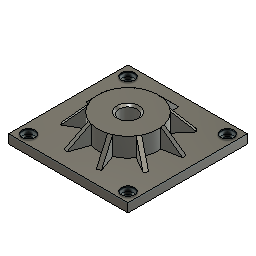
camera_mount (Autodesk Fusion 360 design; units mm, degrees)
Autodesk Fusion 360 part; units mm, degrees
sketch "Sketch1" plane through (0, 0, 0) normal (0, 1, 0) x (1, 0, 0)
  circle A0 centre (0, 0) radius 1.75
  circle A1 centre (50, 0) radius 1.75
  circle A2 centre (0, -50) radius 1.75
  circle A3 centre (50, -50) radius 1.75
  circle A4 centre (25, -25) radius 4.5
  line L0 (-5, 5) -> (55, 5)
  line L1 (55, 5) -> (55, -55)
  line L2 (55, -55) -> (-5, -55)
  line L3 (-5, -55) -> (-5, 5)
  dimension "d1" = 50
  dimension "d2" = 50
  dimension "d3" = 3.5
  dimension "d4" = 3.5
  dimension "d5" = 3.5
  dimension "d6" = 3.5
  dimension "d7" = 9
  constraint coincident A0.centre origin
  constraint horizontal L0
  constraint vertical L1
  constraint horizontal L2
  constraint vertical L3
  measures "d1" distance of A0.centre A2.centre
  measures "d2" distance of A0.centre A1.centre
  measures "d3" diameter of A0
  measures "d4" diameter of A1
  measures "d5" diameter of A2
  measures "d6" diameter of A3
  measures "d7" diameter of A4
extrude "Extrude1" add sketch "Sketch1" along normal blind 4 contours A4 | L0 L1 L2 L3
sketch "Sketch2" plane through (0, 4, 0) normal (0, 1, 0) x (-1, 0, 0)
  circle A0 centre (0, 0) radius 1.75
  circle A1 centre (-50, 0) radius 1.75
  circle A2 centre (0, 50) radius 1.75
  circle A3 centre (-50, 50) radius 1.75
  line L0 (5, 55) -> (-55, 55)
  line L1 (-55, 55) -> (-55, -5)
  line L2 (-55, -5) -> (5, -5)
  line L3 (5, -5) -> (5, 55)
  circle A4 centre (0, 0) radius 3.25
  circle A5 centre (-50, 0) radius 3.25
  circle A6 centre (0, 50) radius 3.25
  circle A7 centre (-50, 50) radius 3.25
  dimension "d10" = 6.5
  dimension "d11" = 6.5
  dimension "d12" = 6.5
  dimension "d13" = 6.5
  constraint concentric A0 A4
  constraint concentric A1 A5
  constraint concentric A2 A6
  constraint concentric A3 A7
  measures "d10" diameter of A4
  measures "d11" diameter of A5
  measures "d12" diameter of A6
  measures "d13" diameter of A7
extrude "Extrude2" add sketch "Sketch2" along normal blind 0.5 contours L0 L1 L2 L3
extrude "Extrude3" cut 1 faces at (-2.7314, 4, -0.2484) along direction (0, -1, 0) blind 2
extrude "Extrude4" cut 1 faces at (-2.7314, 4, 49.7516) along direction (0, -1, 0) blind 2
sketch "Sketch3" plane through (0, 4, 0) normal (0, 1, 0) x (-1, 0, 0)
  circle A0 centre (-50, 0) radius 3.25
  circle A1 centre (-50, 0) radius 1.75
extrude "Extrude5" cut sketch "Sketch3" against normal blind 2
extrude "Extrude6" cut 1 faces at (47.2686, 4, 49.7516) along direction (0, -1, 0) blind 2
sketch "Sketch4" plane through (0, 4.5, 0) normal (0, 1, 0) x (-1, 0, 0)
  circle A0 centre (-50, 50) radius 3.25
  circle A1 centre (-50, 0) radius 3.25
  circle A2 centre (0, 50) radius 3.25
  circle A3 centre (0, 0) radius 3.25
  line L0 (5, -5) -> (5, 55)
  line L1 (5, 55) -> (-55, 55)
  line L2 (-55, 55) -> (-55, -5)
  line L3 (-55, -5) -> (5, -5)
  line L4 (-24, 3) -> (-26, 3)
  line L5 (-10.0926, 8.7898) -> (-11.6247, 7.5042)
  line L6 (-3.1606, 22.1645) -> (-3.5079, 20.1949)
  line L7 (-6.4474, 36.866) -> (-5.4474, 35.134)
  line L8 (-18.4152, 46.0153) -> (-16.5359, 45.3312)
  line L9 (-33.4641, 45.3312) -> (-31.5848, 46.0153)
  line L10 (-44.5526, 35.134) -> (-43.5526, 36.866)
  line L11 (-46.4921, 20.1949) -> (-46.8394, 22.1645)
  line L12 (-38.3753, 7.5042) -> (-39.9074, 8.7898)
  circle A4 centre (-25, 25) radius 15
  line L13 (-11.6247, 7.5042) -> (-16.1457, 12.8921)
  line L14 (-14.6136, 14.1777) -> (-10.0926, 8.7898)
  line L15 (-24, 10.0334) -> (-24, 3)
  line L16 (-26, 3) -> (-26, 10.0334)
  line L17 (-33.8543, 12.8921) -> (-38.3753, 7.5042)
  line L18 (-39.9074, 8.7898) -> (-35.3864, 14.1777)
  line L19 (-39.5656, 21.4163) -> (-46.4921, 20.1949)
  line L20 (-46.8394, 22.1645) -> (-39.9129, 23.3859)
  line L21 (-38.4615, 31.6173) -> (-44.5526, 35.134)
  line L22 (-43.5526, 36.866) -> (-37.4615, 33.3493)
  line L23 (-31.0586, 38.722) -> (-33.4641, 45.3312)
  line L24 (-31.5848, 46.0153) -> (-29.1792, 39.4061)
  line L25 (-20.8208, 39.4061) -> (-18.4152, 46.0153)
  line L26 (-16.5359, 45.3312) -> (-18.9414, 38.722)
  line L27 (-12.5385, 33.3493) -> (-6.4474, 36.866)
  line L28 (-5.4474, 35.134) -> (-11.5385, 31.6173)
  line L29 (-10.0871, 23.3859) -> (-3.1606, 22.1645)
  line L30 (-3.5079, 20.1949) -> (-10.4344, 21.4163)
  line L31 (-25.8167, 5.0167) -> (-26, 3) construction
  arc A5 (-26, 5.025) -> (-25.8167, 5.0167) centre (-25, 25) ccw
  dimension "d27" = 30
  constraint coincident A4 L13.end
  constraint coincident A4 L14.start
  constraint coincident A4 L15.start
  constraint coincident A4 L16.end
  constraint coincident A4 L17.start
  constraint coincident A4 L18.end
  constraint coincident A4 L19.start
  constraint coincident A4 L20.end
  constraint coincident A4 L21.start
  constraint coincident A4 L22.end
  constraint coincident A4 L23.start
  constraint coincident A4 L24.end
  constraint coincident A4 L25.start
  constraint coincident A4 L26.end
  constraint coincident A4 L27.start
  constraint coincident A4 L28.end
  constraint coincident A4 L29.start
  constraint coincident A4 L30.end
  constraint coincident L16 A5.start
  measures "d27" diameter of A4
extrude "Extrude7" add sketch "Sketch4" along normal blind 9.5 contours L4 A4 L15 L16 | A4 | L5 A4 L13 L14 | L12 A4 L17 L18 | L6 A4 L29 L30 | L11 A4 L19 L20 | L10 A4 L21 L22 | L7 A4 L27 L28 | L9 A4 L23 L24 | L8 A4 L25 L26
extrude "Extrude8" add 1 faces at (24.6667, 7.6667, 3) along direction (0, 0, -1) blind 2.5
chamfer "Chamfer1" distance 9.5 angle 45 1 edges at (25, 14, 0.5)
extrude "Extrude9" add 1 faces at (10.6033, 7.6667, 8.3613) along direction (-0.642788, 0, -0.766044) blind 2.5
extrude "Extrude10" add 1 faces at (3.2763, 7.6667, 21.508) along direction (-0.984808, 0, -0.173648) blind 2.5
extrude "Extrude11" add 1 faces at (6.1141, 7.6667, 36.2887) along direction (-0.866025, 0, 0.5) blind 2.5
extrude "Extrude12" add 1 faces at (17.7888, 7.6667, 45.7872) along direction (-0.34202, 0, 0.939693) blind 2.5
extrude "Extrude13" add 1 faces at (32.8377, 7.6667, 45.5592) along direction (0.34202, 0, 0.939693) blind 2.5
extrude "Extrude14" add 1 faces at (44.2192, 7.6667, 35.7113) along direction (0.866025, 0, 0.5) blind 2.5
extrude "Extrude15" add 1 faces at (46.6079, 7.6667, 20.8515) along direction (0.984808, 0, -0.173648) blind 2.5
extrude "Extrude16" add 1 faces at (38.886, 7.6667, 7.9328) along direction (0.642788, 0, -0.766044) blind 2.5
chamfer "Chamfer2" distance 9.5 angle 45 8 edges at (49.1278, 14, 20.7456) (40.7483, 14, 6.2319) (46.2176, 14, 37.25) (9.2517, 14, 6.2319) (33.3795, 14, 48.0225) (16.6205, 14, 48.0225) (3.7824, 14, 37.25) (0.8722, 14, 20.7456)
sketch "Sketch5" plane through (0, 14, 0) normal (0, 1, 0) x (-1, 0, 0)
  line L0 (-10.4015, 21.4105) -> (-10.0542, 23.3801)
  line L1 (-10.0542, 23.3801) -> (-10.0871, 23.3859)
  arc A0 (-10.0871, 23.3859) -> (-11.5385, 31.6173) centre (-25, 25) ccw
  line L2 (-11.5385, 31.6173) -> (-11.5096, 31.634)
  line L3 (-11.5096, 31.634) -> (-12.5096, 33.366)
  line L4 (-12.5096, 33.366) -> (-12.5385, 33.3493)
  arc A1 (-12.5385, 33.3493) -> (-18.9414, 38.722) centre (-25, 25) ccw
  line L5 (-18.9414, 38.722) -> (-18.93, 38.7534)
  line L6 (-18.93, 38.7534) -> (-20.8094, 39.4374)
  line L7 (-20.8094, 39.4374) -> (-20.8208, 39.4061)
  arc A2 (-20.8208, 39.4061) -> (-29.1792, 39.4061) centre (-25, 25) ccw
  line L8 (-29.1792, 39.4061) -> (-29.1906, 39.4374)
  line L9 (-29.1906, 39.4374) -> (-31.07, 38.7534)
  line L10 (-31.07, 38.7534) -> (-31.0586, 38.722)
  arc A3 (-31.0586, 38.722) -> (-37.4615, 33.3493) centre (-25, 25) ccw
  line L11 (-37.4615, 33.3493) -> (-37.4904, 33.366)
  line L12 (-37.4904, 33.366) -> (-38.4904, 31.634)
  line L13 (-38.4904, 31.634) -> (-38.4615, 31.6173)
  arc A4 (-38.4615, 31.6173) -> (-39.9129, 23.3859) centre (-25, 25) ccw
  line L14 (-39.9129, 23.3859) -> (-39.9458, 23.3801)
  line L15 (-39.9458, 23.3801) -> (-39.5985, 21.4105)
  line L16 (-39.5985, 21.4105) -> (-39.5656, 21.4163)
  arc A5 (-39.5656, 21.4163) -> (-35.3864, 14.1777) centre (-25, 25) ccw
  line L17 (-35.3864, 14.1777) -> (-35.4079, 14.1521)
  line L18 (-35.4079, 14.1521) -> (-33.8758, 12.8665)
  line L19 (-33.8758, 12.8665) -> (-33.8543, 12.8921)
  arc A6 (-33.8543, 12.8921) -> (-26, 10.0334) centre (-25, 25) ccw
  line L20 (-26, 10.0334) -> (-26, 10)
  line L21 (-26, 10) -> (-24, 10)
  line L22 (-24, 10) -> (-24, 10.0334)
  arc A7 (-24, 10.0334) -> (-16.1457, 12.8921) centre (-25, 25) ccw
  line L23 (-16.1457, 12.8921) -> (-16.1242, 12.8665)
  line L24 (-16.1242, 12.8665) -> (-14.5921, 14.1521)
  line L25 (-14.5921, 14.1521) -> (-14.6136, 14.1777)
  arc A8 (-14.6136, 14.1777) -> (-10.4344, 21.4163) centre (-25, 25) ccw
  line L26 (-10.4344, 21.4163) -> (-10.4015, 21.4105)
  circle A9 centre (-25, 25) radius 4.5
  dimension "d50" = 9
  constraint concentric A0 A9
  measures "d50" diameter of A9
extrude "Extrude17" cut sketch "Sketch5" against normal blind 12 contours A9
chamfer "Chamfer3" distance 1 angle 45 1 edges at (29.1955, 14, 26.6273)
sketch "Sketch6" plane through (55, 0, 0) normal (1, 0, 0) x (0, 0, -1)
  line L0 (-55, 0) -> (5, 0)
  line L1 (5, 0) -> (5, 4.5)
  line L2 (5, 4.5) -> (-55, 4.5)
  line L3 (-55, 4.5) -> (-55, 0)
